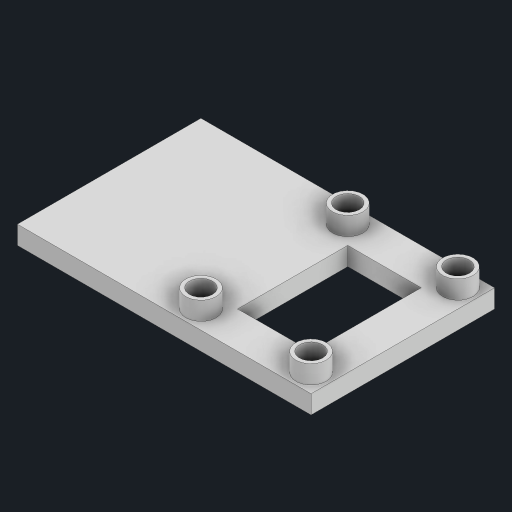
# Autodesk Inventor part: carriage_mount
Saved by Autodesk Inventor 2024 (Build 280153000, 153)
## iProperties
Created: 2024-06-21
Part Number: carriage_mount
Material: Generic
Document SubType Name: Modeling
Designer: mihir
Density: 1 g/cm^3
Appearance: Default
Author: mihir
Autodesk Inventor part; units mm, degrees
ref_plane "YZ Plane" through (0, 0, 0) normal (1, 0, 0) x (0, 1, 0)
ref_plane "XZ Plane" through (0, 0, 0) normal (0, 1, 0) x (-1, 0, 0)
ref_plane "XY Plane" through (0, 0, 0) normal (0, 0, 1) x (1, 0, 0)
sketch "Sketch1" plane through (0, 0, 0) normal (0, 1, 0) x (-1, 0, 0)
  line L0 (0, 0) -> (80, 0)
  line L1 (80, 0) -> (80, -50)
  line L2 (80, -50) -> (0, -50)
  line L3 (0, -50) -> (0, 0)
  line L4 (30, -10) -> (10, -10)
  line L5 (10, -10) -> (10, -40)
  line L6 (10, -40) -> (30, -40)
  line L7 (30, -40) -> (30, -10)
  dimension "d0" = 50
  dimension "d1" = 80
  dimension "d2" = 30
  dimension "d3" = 20
  dimension "d4" = 10
  dimension "d5" = 10
  constraints: 16 end point, 4 parallel, 2 horizontal, 2 perpendicular
  measures "d0" distance of L2.end L0.start
  measures "d1" distance of L0.start L0.end
  measures "d2" distance of L4.end L5.end
  measures "d3" distance of L5.end L6.end
  measures "d4" distance between parallel lines of L2 L6
  measures "d5" distance between parallel lines of L3 L5
extrude "Extrusion1" add sketch "Sketch1" along normal blind 5
sketch "Sketch2" plane through (0, 5, 0) normal (0, 1, 0) x (1, 0, 0)
  line L0 (-10, 40) -> (-10, 10) construction
  line L1 (-10, 10) -> (0, 10) construction
  line L2 (0, 0) -> (0, 50) construction
  line L3 (-5, 5) -> (-5, 10) construction
  line L4 (-10, 10) -> (-30, 10) construction
  line L5 (-10, 10) -> (-10, 0) construction
  line L6 (-80, 0) -> (0, 0) construction
  line L7 (-5, 5) -> (-10, 5) construction
  line L8 (-5, 5) -> (-35, 5) construction
  line L9 (-35, 5) -> (-35, 45) construction
  line L10 (-35, 45) -> (-5, 45) construction
  line L11 (-5, 45) -> (-5, 5) construction
  line L12 (-5, 45) -> (-5, 50) construction
  line L13 (0, 50) -> (-80, 50) construction
  line L14 (-35, 25) -> (-30, 25) construction
  line L15 (-30, 10) -> (-30, 40) construction
  constraints: 20 end point, 4 horizontal, 4 midpoint, 4 vertical, 3 point on line, 2 equal length, 1 perpendicular
hole "Hole1" at (-35, 5, -5) at (-5, 5, -5) at (-35, 5, -45) at (-5, 5, -45) direction (0, -1, 0) diameter 6.3 depth 5 tip angle 118
sketch "Sketch3" plane through (0, 5, 0) normal (0, 1, 0) x (1, 0, 0)
  circle A0 centre (-5, 5) radius 3.15 projected
  circle A1 centre (-5, 5) radius 4.15
  circle A2 centre (-35, 5) radius 3.15 projected
  circle A3 centre (-35, 5) radius 4.15
  circle A4 centre (-35, 45) radius 3.15 projected
  circle A5 centre (-35, 45) radius 4.15
  circle A6 centre (-5, 45) radius 3.15 projected
  circle A7 centre (-5, 45) radius 4.15
  point P0 (0, 0)
  dimension "d15" = 1
  constraints: 4 centre point, 4 coincident, 3 equal radius
  measures "d15" radial gap between concentric circles of A2 A3
extrude "Extrusion2" add sketch "Sketch3" along normal blind 5
equation "\"d0\" = carriage_mount_width"
equation "\"d1\" = carriage_mount_length"
equation "\"d2\" = carriage_mount_cutout_length"
equation "\"d3\" = carriage_mount_cutout_width"
equation "\"d4\" = 0.5 * carriage_mount_width - 0.5 * carriage_mount_cutout_length"
equation "\"d5\" = 0.5 * carriage_mount_width - 0.5 * carriage_mount_cutout_length"
equation "\"d6\" = carriage_mount_thickness"
equation "\"d8\" = rod_diameter + rod_tolerance"
equation "\"d15\" = carriage_mount_wall_thickness"
equation "\"d16\" = carriage_mount_thickness"
equation "\"carriage_mount_length\" = 80"
equation "\"carriage_mount_width\" = 50"
equation "\"carriage_mount_cutout_length\" = 30"
equation "\"carriage_mount_cutout_width\" = 20"
equation "\"screw_diameter\" = 1"
equation "\"rod_diameter\" = 6"
equation "\"rod_tolerance\" = 0.3"
equation "\"carriage_mount_wall_thickness\" = 1"
equation "\"carriage_mount_thickness\" = 5"
body "Solid1"
